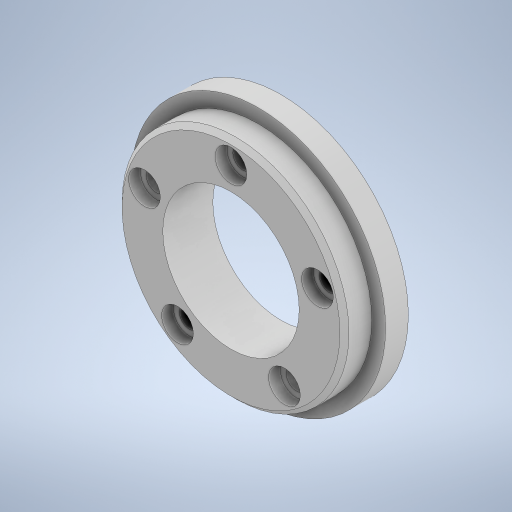
# Autodesk Inventor part: 사이클로이드 기어 축 연결 하우징
Saved by Autodesk Inventor 2023 (Build 270158000, 158)
## iProperties
Created: 2022-06-20
Part Number: 사이클로이드 기어 축 연결 하우징
Material: 일반
Document SubType Name: Modeling
Designer: fly01
Density: 1 g/cm^3
Appearance: 기본값
Author: fly01
Autodesk Inventor part; units mm, degrees
ref_plane "YZ Plane" through (0, 0, 0) normal (1, 0, 0) x (0, 1, 0)
ref_plane "XZ Plane" through (0, 0, 0) normal (0, 1, 0) x (-1, 0, 0)
ref_plane "XY Plane" through (0, 0, 0) normal (0, 0, 1) x (1, 0, 0)
sketch "스케치1" plane through (0, 0, 0) normal (0, 0, 1) x (1, 0, 0)
  circle A0 centre (0, 0) radius 24.95
  circle A1 centre (0, 0) radius 28
  circle A2 centre (0, 0) radius 15
  dimension "d0" = 49.9
  dimension "d1" = 56
  dimension "d2" = 30
  constraints: 3 centre point, 3 coincident
  measures "d0" diameter of A0
  measures "d1" diameter of A1
  measures "d2" diameter of A2
extrude "돌출1" add sketch "스케치1" along normal blind 6 contours A0
extrude "돌출2" add sketch "스케치1" against normal blind 5 contours A0 | A1
sketch "스케치3" plane through (0, 0, 6) normal (0, 0, 1) x (1, 0, 0)
  circle A0 centre (0, 0) radius 20 construction
  circle A1 centre (0, 20) radius 2.2
  circle A2 centre (-19.0211, 6.1803) radius 2.2
  circle A3 centre (-11.7557, -16.1803) radius 2.2
  circle A4 centre (11.7557, -16.1803) radius 2.2
  circle A5 centre (19.0211, 6.1803) radius 2.2
  dimension "d9" = 40
  dimension "d10" = 4.4
  dimension "d13" = 360
  constraints: 5 centre point, 1 coincident, 1 vertical alignment, 13 other
  measures "d10" diameter of A1
extrude "돌출3" cut sketch "스케치3" against normal blind 44.5
sketch "스케치4" plane through (0, 0, -5) normal (0, 0, -1) x (-1, 0, 0)
  circle A0 centre (0, 20) radius 2.2 projected
  line L0 (0, 15.8431) -> (-3.6, 17.9215)
  line L1 (-3.6, 17.9215) -> (-3.6, 22.0785)
  line L2 (-3.6, 22.0785) -> (0, 24.1569)
  line L3 (0, 24.1569) -> (3.6, 22.0785)
  line L4 (3.6, 22.0785) -> (3.6, 17.9215)
  line L5 (3.6, 17.9215) -> (0, 15.8431)
  point P0 (0, 0)
  dimension "d19" = 7.2
  constraints: 12 end point, 1 coincident, 13 other
  measures "d19" distance between parallel lines of L4 L1
extrude "돌출4" cut sketch "스케치4" against normal blind 3.2 contours A0 | L0 L1 L2 L3 L4 L5
pattern_circular "원형 패턴1" count 5 over 360 about axis through (0, 0, 0) along (0, 0, 1) of "돌출4"
sketch "스케치6" plane through (0, 0, 6) normal (0, 0, 1) x (1, 0, 0)
  circle A0 centre (0, 20) radius 2.2 projected
  circle A1 centre (0, 20) radius 3.5
  circle A2 centre (-19.0211, 6.1803) radius 3.5
  circle A3 centre (-11.7557, -16.1803) radius 3.5
  circle A4 centre (11.7557, -16.1803) radius 3.5
  circle A5 centre (19.0211, 6.1803) radius 3.5
  point P0 (0, 0)
  dimension "d26" = 7
  dimension "d29" = 360
  constraints: 5 centre point, 1 coincident, 11 other
  measures "d26" diameter of A1
extrude "돌출5" cut sketch "스케치6" against normal blind 2.6 contours A0 | A1 | A2 | A3 | A4 | A5
chamfer "모따기2" distance 1 angle 45 1 edges at (-24.95, 0, 6)
